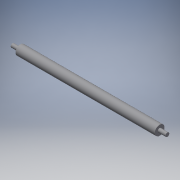
# Autodesk Inventor part: eje
Saved by Autodesk Inventor 2018 (Build 220112000, 112)
## iProperties
Created: 2021-07-05
Part Number: eje
Material: Acero, no aleado
Document SubType Name: Modeling
Designer: GABRIEL
Density: 7.85 g/cm^3
Appearance: Acero
Author: GABRIEL
Autodesk Inventor part; units mm, degrees
ref_plane "YZ Plane" through (0, 0, 0) normal (1, 0, 0) x (0, 1, 0)
ref_plane "XZ Plane" through (0, 0, 0) normal (0, 1, 0) x (-1, 0, 0)
ref_plane "XY Plane" through (0, 0, 0) normal (0, 0, 1) x (1, 0, 0)
sketch "Boceto1" plane through (0, 0, 0) normal (1, 0, 0) x (0, 1, 0)
  circle A0 centre (0, 0) radius 12.5
  circle A1 centre (0, 0) radius 6.75
  dimension "d0" = 25
  dimension "d1" = 13.5
  constraints: 2 centre point, 2 coincident
  measures "d0" diameter of A0
  measures "d1" diameter of A1
extrude "Extrusión1" add sketch "Boceto1" against normal blind 160 contours A1
extrude "Extrusión2" add sketch "Boceto1" along normal mid plane 300
sketch "Boceto2" plane through (0, 0, 0) normal (1, 0, 0) x (0, 0, -1)
  circle A0 centre (0, 0) radius 6.75
  dimension "d6" = 13.5
  constraints: 1 centre point, 1 coincident
  measures "d6" diameter of A0
extrude "Extrusión3" add sketch "Boceto2" along normal blind 180
